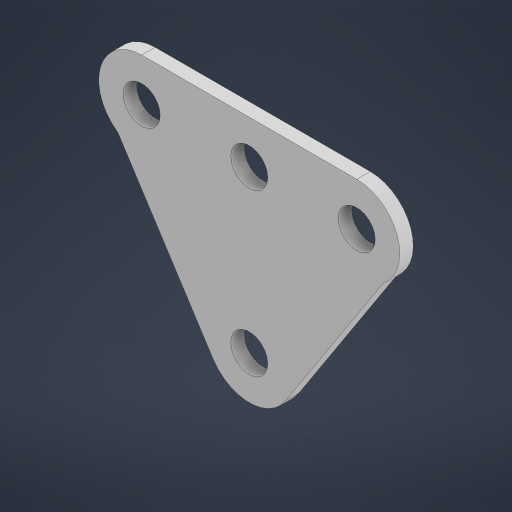
# Autodesk Inventor part: Wing poly connection
Saved by Autodesk Inventor 2023.4 (Build 274418000, 418)
## iProperties
Created: 2024-01-13
Part Number: Wing poly connection
Material: Generic
Document SubType Name: Modeling
Designer: diego
Density: 1 g/cm^3
Appearance: Default
Author: diego
Autodesk Inventor part; units mm, degrees
ref_plane "YZ Plane" through (0, 0, 0) normal (1, 0, 0) x (0, 1, 0)
ref_plane "XZ Plane" through (0, 0, 0) normal (0, 1, 0) x (-1, 0, 0)
ref_plane "XY Plane" through (0, 0, 0) normal (0, 0, 1) x (1, 0, 0)
sketch "Sketch1" plane through (0, 0, 0) normal (0, 0, 1) x (1, 0, 0)
  circle A0 centre (84.4346, 2.8198) radius 2.1844
  line L0 (84.4346, 2.8198) -> (97.1463, 2.8198)
  circle A1 centre (97.1463, 2.8198) radius 2.1844
  line L1 (97.1463, 2.8198) -> (109.8436, 2.8198)
  circle A2 centre (109.8436, 2.8198) radius 2.1844
  circle A3 centre (84.4346, 2.8198) radius 5.08
  circle A4 centre (97.1463, 2.8198) radius 5.08
  circle A5 centre (109.8436, 2.8198) radius 5.08
  line L2 (97.1463, 2.8198) -> (97.1463, -9.8791)
  line L3 (84.4346, 7.8998) -> (97.1463, 7.8998)
  line L4 (109.8436, 7.8998) -> (97.1463, 7.8998)
  line L5 (97.1463, 2.8198) -> (97.1463, -16.2285)
  circle A6 centre (97.1463, -16.2285) radius 5.08
  circle A7 centre (97.1463, -16.2285) radius 2.1844
  line L6 (81.6034, -1.3981) -> (92.8698, -18.9704)
  line L7 (101.4083, -18.9929) -> (112.9486, -1.2008)
  dimension "d46" = 10.16
  dimension "d42" = 4.3688
  dimension "d43" = 4.3688
  dimension "d44" = 4.3688
  dimension "d45" = 10.16
  dimension "d47" = 10.16
  dimension "d50" = 10.16
  dimension "d51" = 4.3688
  constraints: 16 end point, 7 centre point, 7 coincident, 6 point on circle, 4 horizontal, 3 tangent, 2 point on line, 1 collinear, 1 vertical, 1 vertical alignment, 2 other
  measures "d42" diameter of A0
  measures "d43" diameter of A1
  measures "d44" diameter of A2
  measures "d45" diameter of A3
  measures "d47" diameter of A5
  measures "d50" diameter of A6
  measures "d51" diameter of A7
extrude "Extrusion6" add sketch "Sketch1" along normal blind 1.5875 contours A3 L3 A4 L0 | A3 | L0 A4 L2 L5 A6 L6 A3 | A4 L1 A1 L0 | L0 A1 L2 A4 | L4 A5 L1 A4 | L2 A1 L1 A4 | A4 L1 A5 L7 A6 L5 L2 | A6 | A5
body "Solid6"
